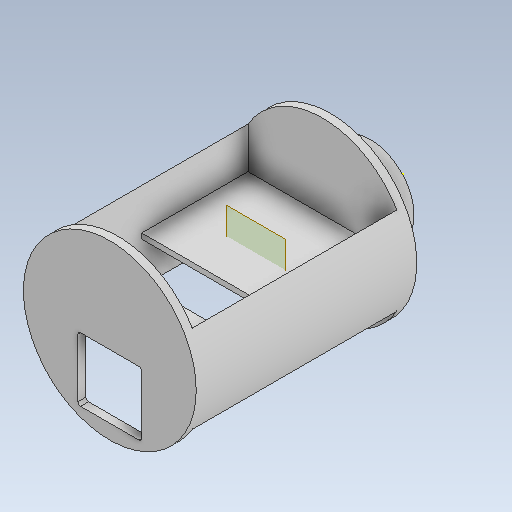
# Autodesk Inventor part: Korpus
Saved by Autodesk Inventor 2020 (Build 240168000, 168)
## iProperties
Created: 2021-10-14
Part Number: Korpus
Material: Ogólny
Document SubType Name: Modeling
Designer: Komputer
Density: 1 g/cm^3
Appearance: Domyślna
Mass: 41.9996 g
Surface Area: 328.715 cm^2
Volume: 41.9996 cm^3
Author: Komputer
Autodesk Inventor part; units mm, degrees
ref_plane "YZ Plane" through (0, 0, 0) normal (1, 0, 0) x (0, 1, 0)
ref_plane "XZ Plane" through (0, 0, 0) normal (0, 1, 0) x (-1, 0, 0)
ref_plane "XY Plane" through (0, 0, 0) normal (0, 0, 1) x (1, 0, 0)
sketch "Szkic1" plane through (0, 0, 0) normal (0, 0, 1) x (1, 0, 0)
  circle A0 centre (0, 0) radius 32.5
  dimension "d0" = 65
  constraints: 1 centre point, 1 coincident
  measures "d0" diameter of A0
extrude "Wyciągnięcie proste1" add sketch "Szkic1" along normal blind 110
ref_plane "Płaszczyzna konstrukcyjna5" through (0, 0, 55) normal (0, 0, -1) x (-1, 0, 0)
sketch "Szkic3" plane through (0, 0, 55) normal (0, 0, -1) x (-1, 0, 0)
  line L0 (0, 0) -> (28, 0)
  line L1 (28, 0) -> (28, 16.5)
  circle A0 centre (0, 0) radius 32.5 projected
  line L2 (28, 0) -> (28, -35.6443)
  line L3 (28, -35.6443) -> (-28, -35.6443)
  line L4 (-28, -35.6443) -> (-28, 35.8328)
  line L5 (-28, 35.8328) -> (28, 35.8328)
  line L6 (28, 35.8328) -> (28, 0)
  dimension "d3" = 28
  dimension "d4" = 56
  dimension "d5" = 56
  constraints: 14 end point, 3 perpendicular, 2 horizontal, 1 point on line, 2 other
  measures "d3" distance of L0.start L0.end
  measures "d4" distance of L2.end L3.end
  measures "d5" distance of L4.end L5.end
extrude "Wyciągnięcie proste2" cut sketch "Szkic3" along normal blind 25 and the other way blind 52 contours L2 A0 L4 L1 | A0 L4 L5 L6 | L2 L3 L4 A0
sketch "Szkic5" plane through (0, 0, 0) normal (0, 0, -1) x (-1, 0, 0)
  circle A0 centre (0, 0) radius 32.5
  constraints: 1 centre point, 1 coincident
extrude "Wyciągnięcie proste3" cut sketch "Szkic5" against normal blind 27
sketch "Szkic6" plane through (0, 0, 27) normal (0, 0, -1) x (-1, 0, 0)
  circle A0 centre (0, 0) radius 15
  circle A1 centre (0, 0) radius 16.5
  dimension "d12" = 30
  dimension "d13" = 33
  constraints: 2 centre point, 2 coincident
  measures "d12" diameter of A0
  measures "d13" diameter of A1
extrude "Wyciągnięcie proste4" add sketch "Szkic6" along normal blind 15
sketch "Szkic7" plane through (0, 0, 27) normal (0, 0, -1) x (-1, 0, 0)
  line L0 (7, -15.9899) -> (-7, -15.9899)
  line L1 (-7, -15.9899) -> (-7, -29.9899)
  line L2 (-7, -29.9899) -> (7, -29.9899)
  line L3 (7, -29.9899) -> (7, -15.9899)
  line L4 (7, -15.9899) -> (-7, -29.9899) construction
  line L5 (-7, -15.9899) -> (7, -29.9899) construction
  point P0 (0, 0)
  point P1 (0, -22.9899)
  dimension "d16" = 14
  dimension "d17" = 14
  constraints: 12 end point, 2 midpoint, 2 parallel, 1 horizontal, 1 perpendicular
  measures "d16" distance of L2.end L1.end
  measures "d17" distance of L1.end L0.end
extrude "Wyciągnięcie proste5" cut sketch "Szkic7" along normal blind 5 and the other way blind 7.5
sketch "Szkic8" plane through (28, -16.5, 107) normal (-1, 0, 0) x (0, 0, 1)
  line L0 (-77, 0) -> (-77, 33) projected
  line L1 (-77, 16.5) -> (-37, 16.5)
  line L2 (0, 0) -> (0, 33) projected
  line L3 (-37, 16.5) -> (-37, 17.5)
  line L4 (-37, 17.5) -> (-37, 15.5)
  line L5 (-37, 15.5) -> (-77, 15.5)
  line L6 (-77, 15.5) -> (-77, 18.2624)
  line L7 (-77, 15.5) -> (-77, 17.5)
  line L8 (-77, 33) -> (-77, 0) projected
  line L9 (-77, 17.5) -> (-37, 17.5)
  line L10 (-20, 18.2624) -> (0, 18.2624)
  line L11 (0, 18.2624) -> (0, 16.2624)
  line L12 (0, 16.2624) -> (-20, 16.2624)
  line L13 (-20, 16.2624) -> (-20, 18.2624)
  point P0 (-107, 16.5)
  dimension "d22" = 40
  dimension "d23" = 1
  dimension "d24" = 2
  dimension "d25" = 2
  dimension "d28" = 2
  dimension "d29" = 20
  constraints: 22 end point, 7 perpendicular, 4 point on line, 1 midpoint, 1 parallel
  measures "d22" distance of L1.start L1.end
  measures "d23" distance of L1.end L3.end
  measures "d24" distance of L3.end L4.end
  measures "d25" distance of L5.end L7.end
  measures "d28" distance of L10.end L11.end
  measures "d29" distance of L11.end L12.end
extrude "Wyciągnięcie proste6" add sketch "Szkic8" along normal blind 56
sketch "Szkic9" plane through (0, 0, 110) normal (0, 0, 1) x (1, 0, 0)
  line L0 (12, -27) -> (-12, -27)
  line L1 (-12, -27) -> (-12, -3)
  line L2 (-12, -3) -> (12, -3)
  line L3 (12, -3) -> (12, -27)
  line L4 (12, -27) -> (-12, -3) construction
  line L5 (-12, -27) -> (12, -3) construction
  point P0 (0, 0)
  point P1 (0, -15)
  dimension "d30" = 24
  dimension "d31" = 24
  constraints: 12 end point, 2 midpoint, 2 parallel, 1 horizontal, 1 perpendicular
  measures "d30" distance of L1.end L2.end
  measures "d31" distance of L0.end L1.end
extrude "Wyciągnięcie proste7" cut sketch "Szkic9" against normal blind 56
fillet "Zaokrąglenie1" radius 1 4 edges at (12, -27, 108.5) (-12, -27, 108.5) (12, -3, 108.5) (-12, -3, 108.5)
sketch "Szkic13" plane through (28, -1, 30) normal (0, -1, 0) x (1, 0, 0)
  point P0 (-28, -30)
